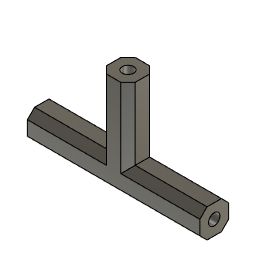
Collin_Support Connector v1 v2 (Autodesk Fusion 360 design; units mm, degrees)
Autodesk Fusion 360 part; units mm, degrees
sketch "Sketch1" plane through (0, 0, 0) normal (0, 1, 0) x (1, 0, 0)
  line L0 (0, 0) -> (24, 0)
  line L1 (24, 0) -> (24, -4)
  line L2 (24, -4) -> (0, -4)
  line L3 (0, -4) -> (0, 0)
  line L4 (10, 0) -> (14, 0)
  line L5 (14, 0) -> (14, -14)
  line L6 (14, -14) -> (10, -14)
  line L7 (10, -14) -> (10, 0)
  dimension "d1" = 24
  dimension "d2" = 4
  dimension "d3" = 24
  dimension "d4" = 4
  dimension "d5" = 4
  dimension "d6" = 10
  dimension "d7" = 10
  constraint horizontal L0
  constraint vertical L1
  constraint horizontal L2
  constraint vertical L3
  constraint horizontal L4
  constraint vertical L5
  constraint horizontal L6
  constraint vertical L7
  constraint coincident L0 L4.start
  measures "d1" distance of L1.end L2.end
  measures "d2" distance of L0.start L2.end
  measures "d3" distance of L0.start L1
  measures "d4" distance of L0.start L2
  measures "d5" distance of L5.end L6.end
  measures "d6" distance of L3 L7
  measures "d7" distance of L2 L6
extrude "Extrude1" add sketch "Sketch1" along normal blind 4
sketch "Sketch2" plane through (24, 0, 0) normal (1, 0, 0) x (0, 1, 0)
  line L0 (0, 4) -> (0, 0)
  line L1 (0, 0) -> (4, 0)
  line L2 (4, 0) -> (4, 4)
  line L3 (4, 4) -> (0, 4)
  circle A0 centre (2, 2) radius 0.8
  dimension "d10" = 1.6
  dimension "d11" = 2
  dimension "d12" = 2
  measures "d10" diameter of A0
  measures "d11" distance of L1 A0.centre
  measures "d12" distance of L0 A0.centre
extrude "Extrude2" cut sketch "Sketch2" against normal blind 24 contours A0
sketch "Sketch3" plane through (0, 0, 14) normal (0, 0, 1) x (-1, 0, 0)
  line L0 (-10, 0) -> (-14, 0)
  line L1 (-14, 0) -> (-14, -4)
  line L2 (-14, -4) -> (-10, -4)
  line L3 (-10, -4) -> (-10, 0)
  circle A0 centre (-12, -2) radius 0.8
  dimension "d15" = 1.6
  dimension "d16" = 2
  dimension "d17" = 2
  measures "d15" diameter of A0
  measures "d16" distance of L3 A0.centre
  measures "d17" distance of L0 A0.centre
extrude "Extrude3" cut sketch "Sketch3" against normal blind 10 contours A0
chamfer "Chamfer1" distance 1 angle 45 10 edges at (19, 0, 4) (14, 0, 9) (10, 0, 9) (5, 0, 4) (12, 0, 0) (19, 4, 4) (14, 4, 9) (10, 4, 9) (5, 4, 4) (12, 4, 0)
equation "d1 = 10 mm + 10 mm + 4 mm"
